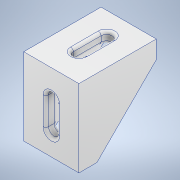
# Autodesk Inventor part: Angulo S
Saved by Autodesk Inventor 2022 (Build 260153000, 153)
## iProperties
Created: 2020-11-04
Part Number: Angulo S
Material: Aluminio 6061
Document SubType Name: Modeling
Designer: Cerberus 1S
Density: 2.7 g/cm^3
Appearance: Aluminio - Plano
Mass: 15.6048 g
Surface Area: 39.5607 cm^2
Volume: 5.77956 cm^3
Author: Cerberus 1S
Autodesk Inventor part; units mm, degrees
ref_plane "YZ Plane" through (0, 0, 0) normal (1, 0, 0) x (0, 1, 0)
ref_plane "XZ Plane" through (0, 0, 0) normal (0, 1, 0) x (-1, 0, 0)
ref_plane "XY Plane" through (0, 0, 0) normal (0, 0, 1) x (1, 0, 0)
sketch "Boceto1" plane through (0, 0, 0) normal (1, 0, 0) x (0, 1, 0)
  line L0 (0, 0) -> (28, 0)
  line L1 (28, 0) -> (28, -28)
  line L2 (28, -28) -> (24, -28)
  line L3 (24, -28) -> (24, -4)
  line L4 (24, -4) -> (0, -4)
  line L5 (0, -4) -> (0, 0)
  dimension "d0" = 28
  dimension "d1" = 28
  dimension "d2" = 4
  dimension "d3" = 4
  constraints: 12 end point, 4 perpendicular, 1 horizontal, 1 parallel
  measures "d0" distance of L0.start L0.end
  measures "d1" distance of L0.end L1.end
  measures "d2" distance between parallel lines of L4 L0
  measures "d3" distance between parallel lines of L1 L3
extrude "Extrusión1" add sketch "Boceto1" along normal blind 20
sketch "Boceto4" plane through (20, 0, 0) normal (1, 0, 0) x (0, 0, -1)
  line L0 (4, 24) -> (28, 24) projected
  line L1 (4, 0) -> (4, 24) projected
  line L2 (28, 24) -> (28, 28) projected
  line L3 (28, 24) -> (28, 21.5)
  line L4 (28, 21.5) -> (6.5, 0)
  line L5 (0, 0) -> (4, 0) projected
  line L6 (6.5, 0) -> (4, 0)
  dimension "d21" = 45
  dimension "d22" = 2.5
  constraints: 6 end point, 1 collinear, 1 vertical
  measures "d21" angle of L1 L4
  measures "d22" distance of L0.end L3.end
extrude "Extrusión4" add sketch "Boceto4" against normal blind 3
sketch "Boceto5" plane through (0, 0, 0) normal (-1, 0, 0) x (0, 0, 1)
  line L0 (-28, 24) -> (-28, 21.5) projected
  line L1 (-28, 21.5) -> (-6.5, 0) projected
  line L2 (-6.5, 0) -> (-4, 0) projected
  line L3 (-4, 24) -> (-4, 0) projected
  line L4 (-28, 24) -> (-4, 24) projected
  point P0 (0, 0)
extrude "Extrusión5" add sketch "Boceto5" against normal blind 3
sketch "Boceto6" plane through (17, 24, -28) normal (0, -1, 0) x (1, 0, 0)
  line L0 (-14, 24) -> (0, 24) projected
  line L1 (-14, 24) -> (0, 24) projected
  line L2 (-7, 24) -> (-7, 0) construction
  line L3 (-14, 0) -> (0, 0) projected
  circle A0 centre (-7, 18) radius 2
  circle A1 centre (-7, 8) radius 2
  line L4 (-17, 28) -> (3, 28) projected
  line L5 (-9, 18) -> (-9, 8)
  line L6 (-5, 8) -> (-5, 18)
  dimension "d27" = 10
  dimension "d28" = 4
  dimension "d29" = 4
  dimension "d30" = 10
  constraints: 6 end point, 4 point on circle, 3 tangent, 2 centre point, 2 midpoint, 2 point on line, 1 parallel
  measures "d27" distance of A1.centre A0.centre
  measures "d28" diameter of A1
  measures "d29" diameter of A0
  measures "d30" distance from line of A0.centre L4
extrude "Extrusión6" cut sketch "Boceto6" against normal through all
fillet "Empalme4" radius 1 8 edges at (10, 24, -22) (8, 24, -15) (10, 24, -8) (12, 24, -15) (10, 28, -8) (8, 28, -15) (10, 28, -22) (12, 28, -15)
sketch "Boceto7" plane through (17, 0, -4) normal (0, 0, -1) x (-1, 0, 0)
  circle A0 centre (7, 8) radius 2
  circle A1 centre (7, 18) radius 2
  line L0 (14, 0) -> (0, 0) projected
  line L1 (9, 18) -> (9, 8)
  line L2 (5, 18) -> (5, 8)
  line L3 (17, 0) -> (-3, 0) projected
  line L4 (7, 0) -> (7, 24) construction
  line L5 (14, 24) -> (0, 24) projected
  dimension "d34" = 4
  dimension "d35" = 4
  dimension "d36" = 10
  dimension "d37" = 8
  constraints: 6 end point, 4 point on circle, 4 tangent, 2 centre point, 2 midpoint, 1 point on line, 1 vertical alignment
  measures "d34" diameter of A0
  measures "d35" diameter of A1
  measures "d36" distance of A0.centre A1.centre
  measures "d37" distance from line of L0 A0.centre
extrude "Extrusión7" cut sketch "Boceto7" against normal through all
fillet "Empalme5" radius 1 8 edges at (8, 13, -4) (10, 6, -4) (12, 13, -4) (10, 20, -4) (10, 20, 0) (12, 13, 0) (10, 6, 0) (8, 13, 0)
